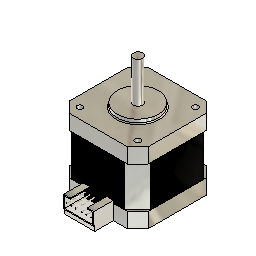
Nema 17 1 to 1 scale (Autodesk Fusion 360 design; units mm, degrees)
Autodesk Fusion 360 part; units mm, degrees
note: some values were not read from the file. Set by a fixed rule: which sketch regions a step uses.
sketch "Sketch1" plane through (0, 0, 0) normal (0, 0, 1) x (1, 0, 0)
  line L0 (21.15, -21.15) -> (-21.15, -21.15)
  line L1 (-21.15, -21.15) -> (-21.15, 21.15)
  line L2 (-21.15, 21.15) -> (21.15, 21.15)
  line L3 (21.15, 21.15) -> (21.15, -21.15)
  line L4 (21.15, -21.15) -> (-21.15, 21.15) construction
  line L5 (-21.15, -21.15) -> (21.15, 21.15) construction
  line L6 (-8.1, -21.15) -> (8.1, -21.15)
  line L7 (-8.1, -21.15) -> (-8.1, -31.15)
  line L8 (-8.1, -31.15) -> (8.1, -31.15)
  line L9 (8.1, -31.15) -> (8.1, -21.15)
  line L10 (15.5, 15.5) -> (-15.5, 15.5) construction
  line L11 (-15.5, 15.5) -> (-15.5, -15.5) construction
  line L12 (-15.5, -15.5) -> (15.5, -15.5) construction
  line L13 (15.5, -15.5) -> (15.5, 15.5) construction
  line L14 (15.5, 15.5) -> (-15.5, -15.5) construction
  line L15 (-15.5, 15.5) -> (15.5, -15.5) construction
  circle A0 centre (-15.5, -15.5) radius 3
  circle A1 centre (15.5, -15.5) radius 3
  line L16 (1.75, 0) -> (22.5, 0)
  circle A2 centre (15.5, 15.5) radius 3
  circle A3 centre (-15.5, 15.5) radius 3
  dimension "d1" = 42.3
  dimension "d2" = 42.3
  dimension "d5" = 10
  dimension "d6" = 16.2
  dimension "d7" = 13.05
  dimension "d23" = 31
  dimension "d24" = 31
  dimension "d25" = 6
  dimension "d26" = 6
  constraint horizontal L0
  constraint perpendicular L0 L1
  constraint parallel L0 L2
  constraint parallel L1 L3
  constraint coincident L4 origin
  constraint coincident L5 origin
  constraint coincident L0 L6.start
  constraint coincident L0 L6.end
  constraint perpendicular L0 L7
  constraint perpendicular L7 L8
  constraint perpendicular L6 L9
  constraint horizontal L10
  constraint perpendicular L10 L11
  constraint parallel L10 L12
  constraint parallel L11 L13
  constraint coincident L14 origin
  constraint coincident L15 origin
  constraint coincident L11.end L12.start
  constraint coincident L12.end L13.start
  constraint symmetric A0 L16 A3
  constraint symmetric A1 L16 A2
  measures "d1" distance of L1.end L2.end
  measures "d2" distance of L0.end L1.end
  measures "d5" distance of L6.start L7.end
  measures "d6" distance of L7.end L8.end
  measures "d7" distance of L3 L9
  measures "d23" distance of L11.end L12.end
  measures "d24" distance of L10.end L11.end
  measures "d25" diameter of A0
  measures "d26" diameter of A1
extrude "Extrude1" add sketch "Sketch1" along normal blind 38 contours L0 L1 L2 L3 L6 | A0 | A1 | A2 | A3
extrude "Extrude2" add sketch "Sketch1" along normal blind 9.4 contours L0 L6 L7 L8 L9
sketch "Sketch2" plane through (0, 0, 38) normal (0, 0, 1) x (-1, 0, 0)
  line L0 (21.15, 21.15) -> (-21.15, 21.15)
  line L1 (-21.15, 21.15) -> (-21.15, -21.15)
  line L2 (-21.15, -21.15) -> (21.15, -21.15)
  line L3 (21.15, -21.15) -> (21.15, 21.15)
  circle A0 centre (0, 0) radius 2.5
  dimension "d12" = 5
  constraint coincident A0.centre origin
  measures "d12" diameter of A0
extrude "Extrude3" add sketch "Sketch2" along normal blind 23.9 contours A0
sketch "Sketch3" plane through (0, 0, 38) normal (0, 0, 1) x (-1, 0, 0)
  circle A0 centre (0, 0) radius 2.5
  line L0 (21.15, 21.15) -> (-21.15, 21.15)
  line L1 (-21.15, 21.15) -> (-21.15, -21.15)
  line L2 (-21.15, -21.15) -> (21.15, -21.15)
  line L3 (21.15, -21.15) -> (21.15, 21.15)
  line L4 (-15.5, 15.5) -> (15.5, 15.5) construction
  line L5 (15.5, 15.5) -> (15.5, -15.5) construction
  line L6 (15.5, -15.5) -> (-15.5, -15.5) construction
  line L7 (-15.5, -15.5) -> (-15.5, 15.5) construction
  line L8 (-15.5, 15.5) -> (15.5, -15.5) construction
  line L9 (15.5, 15.5) -> (-15.5, -15.5) construction
  circle A1 centre (15.5, -15.5) radius 1.5
  circle A2 centre (-15.5, -15.5) radius 1.5
  circle A3 centre (-15.5, 15.5) radius 1.5
  circle A4 centre (15.5, 15.5) radius 1.5
  circle A5 centre (0, 0) radius 11
  dimension "d15" = 31
  dimension "d16" = 31
  dimension "d17" = 3
  dimension "d18" = 3
  dimension "d19" = 3
  dimension "d20" = 3
  dimension "d30" = 22
  constraint horizontal L4
  constraint perpendicular L4 L5
  constraint parallel L4 L6
  constraint parallel L5 L7
  constraint coincident L8 A0.centre
  constraint coincident L9 A0.centre
  constraint coincident A0.centre A5.centre
  constraint coincident L5.end L6.start
  constraint coincident L6.end L7.start
  constraint coincident L4.start L7.end
  constraint coincident L4.end L5.start
  measures "d15" distance of L5.end L6.end
  measures "d16" distance of L4.end L5.end
  measures "d17" diameter of A1
  measures "d18" diameter of A2
  measures "d19" diameter of A3
  measures "d20" diameter of A4
  measures "d30" diameter of A5
extrude "Extrude4" cut sketch "Sketch3" against normal up to surface (38 mm away) contours A1 | A2 | A3 | A4
extrude "Extrude5" cut sketch "Sketch1" along normal blind 3 contours A0 | A1 | A2 | A3
chamfer "Chamfer1" distance 1.5 angle 45 4 edges at (12.703, -16.5848, 3) (-18.297, -16.5848, 3) (12.703, 14.4152, 3) (-18.297, 14.4152, 3)
extrude "Extrude6" add sketch "Sketch3" along normal blind 2.2 contours A5
sketch "Sketch4" plane through (0, 0, 61.9) normal (0, 0, 1) x (-1, 0, 0)
  circle A0 centre (0, 0) radius 2.5
  line L0 (0, 0) -> (2.25, 0)
  line L1 (2.25, 0) -> (2.25, -2.5)
  line L2 (2.25, -2.5) -> (2.25, 0)
  line L3 (2.25, 0) -> (2.25, 2.5)
  dimension "d34" = 2.25
  constraint coincident A0.centre L0.start
  constraint horizontal L0
  constraint perpendicular L0 L1
  constraint perpendicular L0 L3
  measures "d34" distance of A0.centre L0.end
extrude "Extrude7" cut sketch "Sketch4" against normal blind 18 contours A0 L1 L2 L3 picked at (2.4114, -0.0938)
chamfer "Chamfer3" distance 0.5 angle 45 1 edges at (10.2556, -3.9778, 38)
sketch "Sketch5" plane through (0, -31.15, 0) normal (0, -1, 0) x (1, 0, 0)
  line L0 (-8.1, 0) -> (8.1, 0)
  line L1 (8.1, 0) -> (8.1, 9.4)
  line L2 (8.1, 9.4) -> (-8.1, 9.4)
  line L3 (-8.1, 9.4) -> (-8.1, 0)
  line L4 (-8.1, 0) -> (-8.1, 2.6)
  line L5 (-8.1, 2.6) -> (8.1, 2.6)
  line L6 (8.1, 2.6) -> (8.1, 0)
  line L7 (8.1, 0) -> (-8.1, 0)
  line L8 (8.1, 2.6) -> (8.1, 9.4)
  line L9 (8.1, 9.4) -> (4.5, 9.4)
  line L10 (-8.1, 2.6) -> (-8.1, 9.4)
  line L11 (-8.1, 9.4) -> (-4.5, 9.4)
  line L12 (-7.6, 8.9) -> (-4.5, 8.9)
  line L13 (-7.6, 3.1) -> (-7.6, 8.9)
  line L14 (-7.6, 3.1) -> (7.6, 3.1)
  line L15 (7.6, 3.1) -> (7.6, 8.9)
  line L16 (7.6, 8.9) -> (4.5, 8.9)
  line L17 (-4.5, 8.9) -> (-4.5, 9.4)
  line L18 (4.5, 9.4) -> (4.5, 8.9)
  dimension "d38" = 2.6
  dimension "d39" = 3.6
  dimension "d40" = -0.5
  constraint coincident L0.start L3.end
  constraint coincident L3 L4.end
  constraint coincident L1 L5.end
  constraint perpendicular L1 L5
  constraint coincident L0.end L1.start
  constraint coincident L1.end L2.start
  constraint coincident L2 L9.end
  constraint perpendicular L8 L9
  constraint coincident L2.end L3.start
  constraint perpendicular L10 L11
  constraint perpendicular L11 L17
  measures "d38" distance of L0.start L4.end
  measures "d39" distance of L2.end L11.end
extrude "Extrude8" cut sketch "Sketch5" against normal up to surface (10 mm away) contours L2 L12 L13 L14 L15 L16 L17 L18
extrude "Extrude9" add sketch "Sketch5" along normal blind 0.5 contours L1 L2 L3 L5 L8 L9 L10 L11 L12 L13 L14 L15 L16 L17 L18
sketch "Sketch6" plane through (0, -21.15, 0) normal (0, -1, 0) x (1, 0, 0)
  line L0 (21.15, 38) -> (-21.15, 38)
  line L1 (8.1, 0) -> (21.15, 0)
  line L2 (-8.1, 0) -> (-8.1, 9.4)
  line L3 (-8.1, 9.4) -> (-4.5, 9.4)
  line L4 (-4.5, 9.4) -> (-4.5, 8.9)
  line L5 (-4.5, 8.9) -> (-7.6, 8.9)
  line L6 (-7.6, 8.9) -> (-7.6, 3.1)
  line L7 (-7.6, 3.1) -> (7.6, 3.1)
  line L8 (7.6, 3.1) -> (7.6, 8.9)
  line L9 (7.6, 8.9) -> (4.5, 8.9)
  line L10 (4.5, 8.9) -> (4.5, 9.4)
  line L11 (4.5, 9.4) -> (8.1, 9.4)
  line L12 (8.1, 9.4) -> (8.1, 0)
  line L13 (7.6, 3.1) -> (7.6, 8.9)
  line L14 (7.6, 6) -> (6.6, 6) construction
  line L15 (6.6, 6) -> (0, 6) construction
  line L16 (0, 6) -> (3.3, 6) construction
  line L17 (3.3, 6) -> (6.6, 6) construction
  circle A0 centre (6.6, 6) radius 0.25
  line L18 (0, 6) -> (1, 6)
  line L19 (1, 6) -> (6.6, 6) construction
  circle A1 centre (4.125, 6) radius 0.25
  circle A2 centre (1.65, 6) radius 0.25
  line L20 (0, 6) -> (0, 5.2231)
  circle A3 centre (-4.125, 6) radius 0.25
  circle A4 centre (-6.6, 6) radius 0.25
  circle A5 centre (-1.65, 6) radius 0.25
  line L21 (21.15, 0) -> (21.15, 38)
  line L22 (-21.15, 38) -> (-21.15, 0)
  line L23 (-21.15, 0) -> (-8.1, 0)
  dimension "d45" = 1
  dimension "d46" = 0.5
  dimension "d48" = 1
  dimension "d49" = 0.5
  dimension "d50" = 0.5
  dimension "d51" = 2.475
  dimension "d52" = 2.475
  constraint coincident L7.end L8.start
  constraint coincident L8.end L9.start
  constraint midpoint L13 L14.start
  constraint perpendicular L13 L14
  constraint perpendicular L12 L15
  constraint midpoint L15 L16.end
  constraint coincident L14.end L15.start
  constraint coincident L16 L18.end
  constraint midpoint L16 A2.centre
  constraint perpendicular L18 L20
  constraint symmetric A0 L20 A4
  constraint symmetric A1 L20 A3
  constraint symmetric A2 L20 A5
  measures "d45" distance of L14.start L14.end
  measures "d46" diameter of A0
  measures "d48" distance of L15.end L18.end
  measures "d49" diameter of A1
  measures "d50" diameter of A2
  measures "d51" distance of L14.end A1.centre
  measures "d52" distance of A1.centre A2.centre
extrude "Extrude10" add sketch "Sketch6" along normal up to surface (10.5 mm away) contours A0 | A1 | A2 | A3 | A4 | A5
sketch "Sketch7" plane through (0, 21.15, 0) normal (0, 1, 0) x (-1, 0, 0)
  line L0 (-21.15, 0) -> (21.15, 0)
  line L1 (21.15, 0) -> (21.15, 38)
  line L2 (21.15, 38) -> (-21.15, 38)
  line L3 (-21.15, 38) -> (-21.15, 0)
  line L4 (0, 0) -> (0, 8) construction
  line L5 (0, 8) -> (-21.15, 8)
  line L6 (-21.15, 8) -> (-21.15, 0)
  line L7 (0, 8) -> (21.15, 8)
  line L8 (21.15, 8) -> (21.15, 0)
  line L9 (0, 0) -> (0, 38) construction
  line L10 (0, 19) -> (2, 19)
  line L11 (0, 38) -> (0, 30) construction
  line L12 (0, 30) -> (21.15, 30)
  line L13 (21.15, 30) -> (21.15, 38)
  line L14 (0, 30) -> (-21.15, 30)
  line L15 (-21.15, 30) -> (-21.15, 38)
  dimension "d55" = 8
  dimension "d56" = 8
  constraint coincident L4.start L9.start
  constraint perpendicular L0 L4
  constraint coincident L3 L5.end
  constraint perpendicular L3 L5
  constraint coincident L0.start L3.end
  constraint coincident L1 L7.end
  constraint perpendicular L1 L7
  constraint coincident L0.end L1.start
  constraint midpoint L2 L9.end
  constraint midpoint L9 L10.start
  constraint perpendicular L9 L10
  constraint coincident L9 L11.end
  constraint coincident L1 L12.end
  constraint perpendicular L1 L12
  constraint coincident L1.end L2.start
  constraint coincident L3 L14.end
  constraint perpendicular L3 L14
  constraint coincident L2.end L3.start
  measures "d55" distance of L4.start L4.end
  measures "d56" distance of L9.end L11.end
extrude "Extrude11" add sketch "Sketch7" along normal blind 0.01 contours L0 L1 L3 L5 L6 L7 L8 | L1 L2 L3 L12 L13 L14 L15
sketch "Sketch8" plane through (0, -21.15, 0) normal (0, -1, 0) x (1, 0, 0)
  circle A0 centre (-6.6, 6) radius 0.25
  circle A1 centre (4.125, 6) radius 0.25
  circle A2 centre (1.65, 6) radius 0.25
  circle A3 centre (-4.125, 6) radius 0.25
  circle A4 centre (6.6, 6) radius 0.25
  circle A5 centre (-1.65, 6) radius 0.25
  line L0 (-8.1, 0) -> (-8.1, 9.4)
  line L1 (-8.1, 9.4) -> (-4.5, 9.4)
  line L2 (-4.5, 9.4) -> (-4.5, 8.9)
  line L3 (-4.5, 8.9) -> (-7.6, 8.9)
  line L4 (-7.6, 8.9) -> (-7.6, 3.1)
  line L5 (-7.6, 3.1) -> (7.6, 3.1)
  line L6 (7.6, 3.1) -> (7.6, 8.9)
  line L7 (7.6, 8.9) -> (4.5, 8.9)
  line L8 (4.5, 8.9) -> (4.5, 9.4)
  line L9 (4.5, 9.4) -> (8.1, 9.4)
  line L10 (8.1, 9.4) -> (8.1, 0)
  line L11 (8.1, 0) -> (21.15, 0)
  line L12 (21.15, 0) -> (21.15, 38)
  line L13 (21.15, 38) -> (-21.15, 38)
  line L14 (-21.15, 38) -> (-21.15, 0)
  line L15 (-21.15, 0) -> (-8.1, 0)
  line L16 (-21.15, 38) -> (-21.15, 30)
  line L17 (-21.15, 30) -> (21.15, 30)
  line L18 (21.15, 30) -> (21.15, 38)
  line L19 (0, 38) -> (0, 0) construction
  line L20 (0, 0) -> (0, 19) construction
  line L21 (2.7667, 19) -> (0, 19)
  line L22 (-21.15, 0) -> (-21.15, 8)
  line L23 (21.15, 8) -> (21.15, 0)
  line L24 (-21.15, 8) -> (21.15, 8)
  dimension "d59" = 8
  dimension "d60" = 8
  constraint coincident L13.end L14.start
  constraint perpendicular L13 L16
  constraint coincident L12 L17.end
  constraint perpendicular L12 L17
  constraint coincident L12.end L13.start
  constraint midpoint L13 L19.start
  constraint coincident L19.end L20.start
  constraint midpoint L19 L20.end
  constraint perpendicular L19 L21
  constraint coincident L14.end L15.start
  constraint coincident L14 L22.end
  constraint perpendicular L15 L22
  constraint coincident L12 L23.start
  constraint coincident L11.end L12.start
  constraint perpendicular L23 L24
  measures "d59" distance of L13.end L16.end
  measures "d60" distance of L23.start L11.end
extrude "Extrude12" add sketch "Sketch8" along normal blind 0.01 contours L0 L14 L15 L22 L24 | L12 L13 L14 L16 L17 L18 | L10 L11 L12 L23 L24
sketch "Sketch9" plane through (21.15, 0, 0) normal (1, 0, 0) x (0, 1, 0)
  line L0 (-21.16, 0) -> (21.16, 0)
  line L1 (21.16, 0) -> (21.16, 8)
  line L2 (21.16, 8) -> (21.15, 8)
  line L3 (21.15, 8) -> (21.15, 30)
  line L4 (21.15, 30) -> (21.16, 30)
  line L5 (21.16, 30) -> (21.16, 38)
  line L6 (21.16, 38) -> (-21.16, 38)
  line L7 (-21.16, 38) -> (-21.16, 30)
  line L8 (-21.16, 30) -> (-21.15, 30)
  line L9 (-21.15, 30) -> (-21.15, 8)
  line L10 (-21.15, 8) -> (-21.16, 8)
  line L11 (-21.16, 8) -> (-21.16, 0)
  line L12 (21.16, 30) -> (-21.16, 30)
  line L13 (-21.16, 8) -> (21.15, 8)
  constraint coincident L4.end L5.start
  constraint coincident L7.end L8.start
  constraint coincident L10.end L11.start
  constraint coincident L2.end L3.start
sketch "Sketch10" plane through (-21.15, 0, 0) normal (-1, 0, 0) x (0, -1, 0)
  line L0 (-21.16, 0) -> (21.16, 0)
  line L1 (21.16, 0) -> (21.16, 8)
  line L2 (21.16, 8) -> (21.15, 8)
  line L3 (21.15, 8) -> (21.15, 30)
  line L4 (21.15, 30) -> (21.16, 30)
  line L5 (21.16, 30) -> (21.16, 38)
  line L6 (21.16, 38) -> (-21.16, 38)
  line L7 (-21.16, 38) -> (-21.16, 30)
  line L8 (-21.16, 30) -> (-21.15, 30)
  line L9 (-21.15, 30) -> (-21.15, 8)
  line L10 (-21.15, 8) -> (-21.16, 8)
  line L11 (-21.16, 8) -> (-21.16, 0)
  line L12 (21.15, 30) -> (-21.16, 30)
  line L13 (-21.15, 8) -> (21.16, 8)
  constraint coincident L3.end L4.start
  constraint coincident L7.end L8.start
  constraint coincident L9.end L10.start
  constraint coincident L1.end L2.start
extrude "Extrude13" cut sketch "Sketch10" against normal blind 0.01 contours L3 L9 L12 L13
extrude "Extrude14" cut sketch "Sketch9" against normal blind 0.01 contours L3 L9 L12 L13
chamfer "Chamfer4" distance 7 angle 45 1 edges at (-21.14, -21.15, 19)
chamfer "Chamfer5" distance 7 angle 45 3 edges at (21.14, -21.15, 19) (21.14, 21.15, 19) (-21.14, 21.15, 19)
chamfer "Chamfer6" distance 5.5 angle 45 8 edges at (-21.15, 21.16, 4) (-21.15, -21.16, 4) (-21.15, -21.16, 34) (-21.15, 21.16, 34) (21.15, 21.16, 4) (21.15, -21.16, 4) (21.15, -21.16, 34) (21.15, 21.16, 34)
